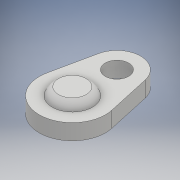
# Autodesk Inventor part: Stylis holder
Saved by Autodesk Inventor 2017 (Build 210142000, 142)
## iProperties
Created: 2017-05-05
Part Number: Stylis holder
Material: Generic
Document SubType Name: Modeling
Designer: andrew
Density: 1 g/cm^3
Appearance: Default
Author: andrew
Autodesk Inventor part; units mm, degrees
ref_plane "YZ Plane" through (0, 0, 0) normal (1, 0, 0) x (0, 1, 0)
ref_plane "XZ Plane" through (0, 0, 0) normal (0, 1, 0) x (-1, 0, 0)
ref_plane "XY Plane" through (0, 0, 0) normal (0, 0, 1) x (1, 0, 0)
sketch "Sketch1" plane through (0, 0, 0) normal (0, 0, 1) x (1, 0, 0)
  circle A0 centre (-0.0198, -0.0084) radius 1.4858
  arc A1 (0.0044, -3.1481) -> (0.0044, -8.2481) centre (0.0044, -5.6981) ccw construction
  arc A2 (0.0044, -8.2481) -> (0.0044, -3.1481) centre (0.0044, -5.6981) ccw construction
  line L0 (-5.8056, -3.1481) -> (0.0044, -3.1481) construction
  line L1 (0.0044, -8.2481) -> (-5.8056, -8.2481) construction
  line L2 (2.5544, -5.6981) -> (5.0544, -5.6981) construction
  line L3 (-5.8056, -3.1481) -> (-5.8056, -8.2481) construction
  arc A3 (2.9095, 0.6389) -> (-2.9546, 0.6139) centre (-0.0198, -0.0084) ccw
  arc A4 (-4.1081, -4.8261) -> (4.1094, -4.7911) centre (0.0044, -5.6981) ccw
  line L4 (2.9095, 0.6389) -> (4.1094, -4.7911)
  line L5 (-2.9546, 0.6139) -> (-4.1081, -4.8261)
  point P0 (0, 0)
  dimension "d0" = 2.5
  dimension "d1" = 6
  constraints: 12 end point, 9 point on circle, 5 centre point, 5 tangent, 2 coincident, 1 horizontal, 1 vertical
  measures "d0" distance of L2.start L2.end
  measures "d1" diameter of A3
extrude "Extrusion1" add sketch "Sketch1" along normal blind 2
sketch "Sketch2" plane through (0, 0, 2) normal (0, 0, 1) x (1, 0, 0)
  circle A0 centre (-0.0198, -0.0084) radius 1.4858
  arc A1 (0.0044, -3.1481) -> (0.0044, -8.2481) centre (0.0044, -5.6981) ccw construction
  arc A2 (0.0044, -8.2481) -> (0.0044, -3.1481) centre (0.0044, -5.6981) ccw construction
  line L0 (-5.8056, -3.1481) -> (0.0044, -3.1481) construction
  line L1 (0.0044, -8.2481) -> (-5.8056, -8.2481) construction
  line L2 (2.5544, -5.6981) -> (5.0544, -5.6981) construction
  line L3 (-5.8056, -3.1481) -> (-5.8056, -8.2481) construction
  arc A3 (2.9095, 0.6389) -> (-2.9546, 0.6139) centre (-0.0198, -0.0084) ccw
  arc A4 (-4.1081, -4.8261) -> (4.1094, -4.7911) centre (0.0044, -5.6981) ccw
  line L4 (2.9095, 0.6389) -> (4.1094, -4.7911)
  line L5 (-2.9546, 0.6139) -> (-4.1081, -4.8261)
  circle A5 centre (0.0044, -5.6981) radius 2.55
  point P0 (0, 0)
  point P1 (0, 0)
  dimension "d4" = 2.5
  dimension "d5" = 6
  constraints: 12 end point, 9 point on circle, 6 centre point, 5 tangent, 3 coincident, 1 concentric, 1 horizontal, 1 vertical
  measures "d4" distance of L2.start L2.end
  measures "d5" diameter of A3
extrude "Extrusion2" add sketch "Sketch2" along normal blind 1.5 contours A5
fillet "Fillet1" radius 2.5 1 edges at (-2.5456, -5.6981, 3.5)
sketch "Sketch3" plane through (2.9095, 0.6389, 2) normal (0.9764456, 0.2157637, 0) x (0, 0, -1)
  line L0 (0, 3) -> (0, 0) projected
  line L1 (0, 0) -> (-1, 0)
  line L2 (-1, 0) -> (-1, -8.6875)
  line L3 (-1, -8.6875) -> (-2.9665, -8.6875)
  line L4 (-2.9665, -8.6875) -> (-2.9665, 0)
  line L5 (-2.9665, 0) -> (-1, 0)
  point P0 (2, 0.0039)
  point P1 (0, 1.2408)
  dimension "d9" = 1
  constraints: 10 end point, 4 perpendicular, 1 horizontal, 1 point on line
  measures "d9" distance of L0.end L1.end
extrude "Extrusion3" cut sketch "Sketch3" against normal blind 10
body "Solid1"
